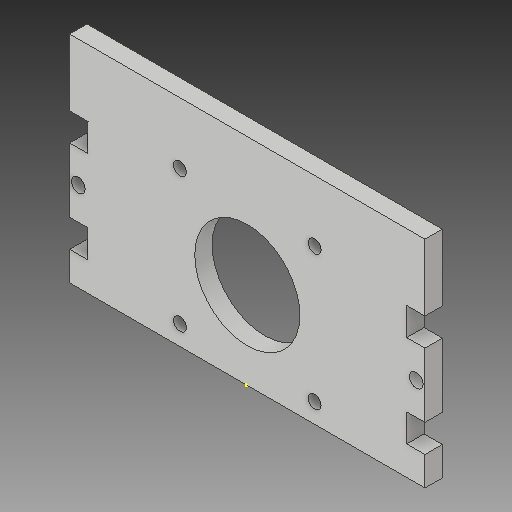
# Autodesk Inventor part: Motor_brace_2
Saved by Autodesk Inventor 2019 (Build 230136000, 136)
## iProperties
Created: 2020-03-11
Part Number: Motor_brace_2
Material: Generic
Document SubType Name: Modeling
Designer: Vijay
Density: 1 g/cm^3
Appearance: Default
Author: Vijay
Autodesk Inventor part; units mm, degrees
ref_plane "YZ Plane" through (0, 0, 0) normal (1, 0, 0) x (0, 1, 0)
ref_plane "XZ Plane" through (0, 0, 0) normal (0, 1, 0) x (-1, 0, 0)
ref_plane "XY Plane" through (0, 0, 0) normal (0, 0, 1) x (1, 0, 0)
sketch "Sketch1" plane through (0, 0, 0) normal (0, 0, 1) x (1, 0, 0)
  line L0 (20, 35.0868) -> (15.0858, 40.001) construction
  line L1 (15.0858, 40.001) -> (-15.0858, 40.001) construction
  line L2 (-15.0858, 40.001) -> (-20, 35.0868) construction
  line L3 (-20, 35.0868) -> (-20, 4.9152) construction
  line L4 (-20, 4.9152) -> (-15.0858, 0.001) construction
  line L5 (-15.0858, 0.001) -> (15.0858, 0.001) construction
  line L6 (15.0858, 0.001) -> (20, 4.9152) construction
  line L7 (20, 4.9152) -> (20, 35.0868) construction
  spline S0 degree 3 number of poles 98 construction
  spline S1 degree 3 number of poles 98 construction
  spline S2 degree 3 number of poles 98 construction
  spline S3 degree 3 number of poles 98 construction
  circle A0 centre (0, 20.001) radius 11 construction
  spline S4 degree 3 number of poles 98 construction
  spline S5 degree 3 number of poles 98 construction
  spline S6 degree 3 number of poles 98 construction
  spline S7 degree 3 number of poles 98 construction
  line L8 (-152.3368, 49.5885) -> (152.3133, 49.5884) construction
  line L9 (-40.8871, 0.001) -> (40.8871, 0.001)
  line L10 (40.8871, 0.001) -> (40.8871, 40.001)
  line L11 (40.8871, 40.001) -> (-40.8871, 40.001)
  line L12 (-40.8871, 40.001) -> (-40.8871, 0.001)
  line L13 (-40.8871, 0.001) -> (40.8871, 40.001) construction
  line L14 (40.8871, 0.001) -> (-40.8871, 40.001) construction
  line L15 (40.8871, 40.001) -> (-40.8871, 40.001)
  line L16 (-40.8871, 40.001) -> (-40.8871, 49.5885)
  line L17 (-40.8871, 49.5885) -> (40.8871, 49.5885)
  line L18 (40.8871, 49.5885) -> (40.8871, 40.001)
  circle A1 centre (15.5, 4.501) radius 1.5
  circle A2 centre (-15.5, 4.501) radius 1.5
  circle A3 centre (-15.5, 35.501) radius 1.5
  circle A4 centre (15.5, 35.501) radius 1.5
  circle A5 centre (0, 20.001) radius 12.0934
  point P0 (0, 0)
  constraints: 20 end point, 4 parallel, 2 horizontal, 2 midpoint, 2 perpendicular, 1 centre point, 1 coincident, 1 point on line
extrude "Extrusion1" add sketch "Sketch1" along normal blind 4
sketch "Sketch2" plane through (0, 0, 4) normal (0, 0, 1) x (1, 0, 0)
  line L0 (36.8871, 28.0768) -> (36.8871, 34.0768) construction
  line L1 (36.8871, 28.0768) -> (40.8871, 28.0768) construction
  line L2 (40.8871, 34.0768) -> (40.8871, 28.0768) construction
  line L3 (36.8871, 34.0768) -> (40.8871, 34.0768) construction
  line L4 (36.8871, 6.8768) -> (36.8871, 12.8768) construction
  line L5 (36.8871, 6.8768) -> (40.8871, 6.8768) construction
  line L6 (40.8871, 12.8768) -> (40.8871, 6.8768) construction
  line L7 (36.8871, 12.8768) -> (40.8871, 12.8768) construction
  line L8 (-40.8871, 28.0768) -> (-40.8871, 34.0768) construction
  line L9 (-40.8871, 28.0768) -> (-36.8871, 28.0768) construction
  line L10 (-36.8871, 34.0768) -> (-36.8871, 28.0768) construction
  line L11 (-40.8871, 34.0768) -> (-36.8871, 34.0768) construction
  line L12 (-40.8871, 6.8768) -> (-40.8871, 12.8768) construction
  line L13 (-40.8871, 6.8768) -> (-36.8871, 6.8768) construction
  line L14 (-36.8871, 12.8768) -> (-36.8871, 6.8768) construction
  line L15 (-40.8871, 12.8768) -> (-36.8871, 12.8768) construction
  line L16 (-40.8871, 18.9768) -> (-40.8871, 21.9768) construction
  line L17 (-40.8871, 18.9768) -> (-36.8871, 18.9768) construction
  line L18 (-36.8871, 21.9768) -> (-36.8871, 18.9768) construction
  line L19 (-40.8871, 21.9768) -> (-36.8871, 21.9768) construction
  line L20 (36.8871, 18.9768) -> (36.8871, 21.9768) construction
  line L21 (36.8871, 18.9768) -> (40.8871, 18.9768) construction
  line L22 (40.8871, 21.9768) -> (40.8871, 18.9768) construction
  line L23 (36.8871, 21.9768) -> (40.8871, 21.9768) construction
  circle A0 centre (-38.8871, 20.4768) radius 1.6
  circle A1 centre (38.8871, 20.4768) radius 1.6
  line L24 (-36.6871, 34.2768) -> (-36.6871, 27.8768)
  line L25 (-36.6871, 27.8768) -> (-41.0871, 27.8768)
  line L26 (-41.0871, 27.8768) -> (-41.0871, 34.2768)
  line L27 (-41.0871, 34.2768) -> (-36.6871, 34.2768)
  line L28 (-36.6871, 13.0768) -> (-36.6871, 6.6768)
  line L29 (-36.6871, 6.6768) -> (-41.0871, 6.6768)
  line L30 (-41.0871, 6.6768) -> (-41.0871, 13.0768)
  line L31 (-41.0871, 13.0768) -> (-36.6871, 13.0768)
  line L32 (41.0871, 34.2768) -> (41.0871, 27.8768)
  line L33 (41.0871, 27.8768) -> (36.6871, 27.8768)
  line L34 (36.6871, 27.8768) -> (36.6871, 34.2768)
  line L35 (36.6871, 34.2768) -> (41.0871, 34.2768)
  line L36 (41.0871, 13.0768) -> (41.0871, 6.6768)
  line L37 (41.0871, 6.6768) -> (36.6871, 6.6768)
  line L38 (36.6871, 6.6768) -> (36.6871, 13.0768)
  line L39 (36.6871, 13.0768) -> (41.0871, 13.0768)
  point P0 (0, 0)
  dimension "d2" = 3.2
  dimension "d3" = 3.2
  dimension "d4" = 0.2
  dimension "d5" = 0.2
  dimension "d6" = 0.2
  dimension "d7" = 0.2
  constraints: 32 end point, 2 centre point, 12 other
  measures "d2" diameter of A0
  measures "d3" diameter of A1
  measures "d4" distance between parallel lines of L11 L27
  measures "d5" distance between parallel lines of L15 L31
  measures "d6" distance between parallel lines of L3 L35
  measures "d7" distance between parallel lines of L7 L39
extrude "Extrusion2" cut sketch "Sketch2" against normal through all
sketch "Sketch3" plane through (0, 0, 4) normal (0, 0, 1) x (1, 0, 0)
  point P0 (0, 0)
body "Solid1"
